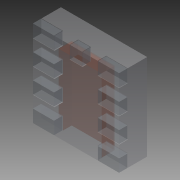
# Autodesk Inventor part: Si1143
Saved by Autodesk Inventor 2013 (Build 170138000, 138)
## iProperties
Created: 2015-06-30
Part Number: Si1143
Material: Ogólny
Document SubType Name: Modeling
Designer: terg
Density: 1 g/cm^3
Author: terg
Autodesk Inventor part; units mm, degrees
ref_plane "YZ Plane" through (0, 0, 0) normal (1, 0, 0) x (0, 1, 0)
ref_plane "XZ Plane" through (0, 0, 0) normal (0, 1, 0) x (-1, 0, 0)
sketch "Szkic1" plane through (0, 0, 0) normal (0, 1, 0) x (-1, 0, 0)
  line L0 (0, 0) -> (2, 0)
  line L1 (2, 0) -> (2, 2)
  line L2 (2, 2) -> (0, 2)
  line L3 (0, 2) -> (0, 0)
  dimension "d0" = 2
  dimension "d1" = 2
  constraints: 8 end point, 2 parallel, 1 horizontal, 1 perpendicular
  measures "d0" distance of L2.end L1.end
  measures "d1" distance of L1.end L0.end
extrude "Wyciągnięcie proste1" add sketch "Szkic1" along normal blind 0.65
sketch "Szkic2" plane through (0, 0, 0) normal (0, -1, 0) x (1, 0, 0)
  line L0 (0, 2) -> (0, 0) projected
  line L1 (-2, 2) -> (0, 2) projected
  line L2 (-2, 0) -> (-2, 2) projected
  line L3 (0, 0) -> (-0.5, 0)
  line L4 (-0.5, 0) -> (-0.5, 0.3)
  line L5 (-0.5, 0.3) -> (0, 0.3)
  line L6 (0, 0.3) -> (0, 0)
  line L7 (0, 0.5667) -> (-0.5, 0.5667)
  line L8 (-0.5, 0.5667) -> (-0.5, 0.8667)
  line L9 (-0.5, 0.8667) -> (0, 0.8667)
  line L10 (0, 0.8667) -> (0, 0.5667)
  line L11 (0, 1.1333) -> (-0.5, 1.1333)
  line L12 (-0.5, 1.1333) -> (-0.5, 1.4333)
  line L13 (-0.5, 1.4333) -> (0, 1.4333)
  line L14 (0, 1.4333) -> (0, 1.1333)
  line L15 (0, 1.7) -> (-0.5, 1.7)
  line L16 (-0.5, 1.7) -> (-0.5, 2)
  line L17 (-0.5, 2) -> (0, 2)
  line L18 (0, 2) -> (0, 1.7)
  line L19 (-2, 0) -> (-1.5, 0)
  line L20 (-1.5, 0) -> (-1.5, 0.3)
  line L21 (-1.5, 0.3) -> (-2, 0.3)
  line L22 (-2, 0.3) -> (-2, 0)
  line L23 (-2, 0.5667) -> (-1.5, 0.5667)
  line L24 (-1.5, 0.5667) -> (-1.5, 0.8667)
  line L25 (-1.5, 0.8667) -> (-2, 0.8667)
  line L26 (-2, 0.8667) -> (-2, 0.5667)
  line L27 (-2, 1.1333) -> (-1.5, 1.1333)
  line L28 (-1.5, 1.1333) -> (-1.5, 1.4333)
  line L29 (-1.5, 1.4333) -> (-2, 1.4333)
  line L30 (-2, 1.4333) -> (-2, 1.1333)
  line L31 (-2, 1.7) -> (-1.5, 1.7)
  line L32 (-1.5, 1.7) -> (-1.5, 2)
  line L33 (-1.5, 2) -> (-2, 2)
  line L34 (-2, 2) -> (-2, 1.7)
  line L35 (-0.85, 2) -> (-1.15, 2)
  line L36 (-1.15, 2) -> (-1.15, 1.7)
  line L37 (-1.15, 1.7) -> (-0.85, 1.7)
  line L38 (-0.85, 1.7) -> (-0.85, 2)
  dimension "d4" = 0.5
  dimension "d5" = 0.3
  dimension "d6" = 0.5
  dimension "d7" = 0.3
  dimension "d8" = 0.5
  dimension "d9" = 0.3
  dimension "d10" = 0.5
  dimension "d11" = 0.3
  dimension "d12" = 0
  dimension "d13" = 0.2667
  dimension "d14" = 0.2667
  dimension "d15" = 0.2667
  dimension "d16" = 0.5
  dimension "d17" = 0.3
  dimension "d18" = 0.5
  dimension "d19" = 0.3
  dimension "d20" = 0.5
  dimension "d21" = 0.3
  dimension "d22" = 0.5
  dimension "d23" = 0.3
  dimension "d24" = 0
  dimension "d25" = 0.2667
  dimension "d26" = 0.2667
  dimension "d27" = 0.3
  dimension "d28" = 0.3
  dimension "d29" = 0.85
  dimension "d30" = 0.85
  constraints: 72 end point, 19 equal length, 9 horizontal, 9 perpendicular, 7 point on line
  measures "d4" distance of L4.end L5.end
  measures "d5" distance of L3.end L4.end
  measures "d6" distance of L8.end L9.end
  measures "d7" distance of L7.end L8.end
  measures "d8" distance of L12.end L13.end
  measures "d9" distance of L11.end L12.end
  measures "d10" distance of L16.end L17.end
  measures "d11" distance of L15.end L16.end
  measures "d12" distance between parallel lines of L1 L17
  measures "d13" distance between parallel lines of L13 L15
  measures "d14" distance between parallel lines of L9 L11
  measures "d15" distance between parallel lines of L5 L7
  measures "d16" distance of L21.end L20.end
  measures "d17" distance of L20.end L19.end
  measures "d18" distance of L25.end L24.end
  measures "d19" distance of L24.end L23.end
  measures "d20" distance of L29.end L28.end
  measures "d21" distance of L28.end L27.end
  measures "d22" distance of L33.end L32.end
  measures "d23" distance of L32.end L31.end
  measures "d24" distance between parallel lines of L15 L31
  measures "d25" distance between parallel lines of L21 L23
  measures "d26" distance between parallel lines of L27 L25
  measures "d27" distance of L37.end L36.end
  measures "d28" distance of L36.end L35.end
  measures "d29" distance between parallel lines of L2 L36
  measures "d30" distance between parallel lines of L0 L38
extrude "Wyciągnięcie proste2" cut sketch "Szkic2" against normal blind 0.2
sketch "Szkic4" plane through (0, 0, 0) normal (0, -1, 0) x (1, 0, 0)
  line L0 (-1.5, 0.5667) -> (-2, 0.5667) projected
  line L1 (-2, 0.3) -> (-2, 0.5667) projected
  line L2 (-2, 0.3) -> (-1.5, 0.3) projected
  line L3 (-1.5, 0.3) -> (-1.5, 0) projected
  line L4 (-0.5, 0) -> (-1.5, 0) projected
  line L5 (-0.5, 0) -> (-0.5, 0.3) projected
  line L6 (-0.5, 0.3) -> (0, 0.3) projected
  line L7 (0, 0.5667) -> (-0.5, 0.5667) projected
  line L8 (-0.5, 0.5667) -> (-0.5, 0.8667) projected
  line L9 (-0.5, 0.8667) -> (0, 0.8667) projected
  line L10 (0, 1.1333) -> (-0.5, 1.1333) projected
  line L11 (-0.5, 1.1333) -> (-0.5, 1.4333) projected
  line L12 (-0.5, 1.4333) -> (0, 1.4333) projected
  line L13 (0, 1.7) -> (0, 1.4333) projected
  line L14 (0, 1.7) -> (-0.5, 1.7) projected
  line L15 (-0.5, 1.7) -> (-0.5, 2) projected
  line L16 (-0.85, 2) -> (-0.5, 2) projected
  line L17 (-0.85, 2) -> (-0.85, 1.7) projected
  line L18 (-0.85, 1.7) -> (-1.15, 1.7) projected
  line L19 (-1.15, 1.7) -> (-1.15, 2) projected
  line L20 (-1.5, 2) -> (-1.15, 2) projected
  line L21 (-1.5, 2) -> (-1.5, 1.7) projected
  line L22 (-1.5, 1.7) -> (-2, 1.7) projected
  line L23 (-2, 1.4333) -> (-2, 1.7) projected
  line L24 (-2, 1.4333) -> (-1.5, 1.4333) projected
  line L25 (-1.5, 1.4333) -> (-1.5, 1.1333) projected
  line L26 (-1.5, 1.1333) -> (-2, 1.1333) projected
  line L27 (-2, 0.8667) -> (-1.5, 0.8667) projected
  line L28 (-1.5, 0.8667) -> (-1.5, 0.5667) projected
  line L29 (-1.51, 1.71) -> (-2, 1.71)
  line L30 (-2, 1.71) -> (-2, 2)
  line L31 (-2, 2) -> (-1.51, 2)
  line L32 (-1.51, 2) -> (-1.51, 1.71)
  line L33 (-2, 1.4233) -> (-1.51, 1.4233)
  line L34 (-1.51, 1.4233) -> (-1.51, 1.1433)
  line L35 (-1.51, 1.1433) -> (-2, 1.1433)
  line L36 (-2, 1.1433) -> (-2, 1.4233)
  line L37 (-2, 0.8567) -> (-1.51, 0.8567)
  line L38 (-1.51, 0.8567) -> (-1.51, 0.5767)
  line L39 (-1.51, 0.5767) -> (-2, 0.5767)
  line L40 (-2, 0.5767) -> (-2, 0.8567)
  line L41 (-2, 0.29) -> (-1.51, 0.29)
  line L42 (-1.51, 0.29) -> (-1.51, 0)
  line L43 (-1.51, 0) -> (-2, 0)
  line L44 (-2, 0) -> (-2, 0.29)
  line L45 (-0.49, 0.29) -> (0, 0.29)
  line L46 (0, 0.29) -> (0, 0)
  line L47 (0, 0) -> (-0.49, 0)
  line L48 (-0.49, 0) -> (-0.49, 0.29)
  line L49 (-0.49, 0.8567) -> (0, 0.8567)
  line L50 (0, 0.8567) -> (0, 0.5767)
  line L51 (0, 0.5767) -> (-0.49, 0.5767)
  line L52 (-0.49, 0.5767) -> (-0.49, 0.8567)
  line L53 (-0.49, 1.4233) -> (0, 1.4233)
  line L54 (0, 1.4233) -> (0, 1.1433)
  line L55 (0, 1.1433) -> (-0.49, 1.1433)
  line L56 (-0.49, 1.1433) -> (-0.49, 1.4233)
  line L57 (-0.49, 2) -> (0, 2)
  line L58 (0, 2) -> (0, 1.71)
  line L59 (0, 1.71) -> (-0.49, 1.71)
  line L60 (-0.49, 1.71) -> (-0.49, 2)
  line L61 (-1.14, 2) -> (-0.86, 2)
  line L62 (-0.86, 2) -> (-0.86, 1.71)
  line L63 (-0.86, 1.71) -> (-1.14, 1.71)
  line L64 (-1.14, 1.71) -> (-1.14, 2)
  dimension "d33" = 0.01
  dimension "d34" = 0.01
  dimension "d35" = 0
  dimension "d36" = 0
  dimension "d37" = 0.01
  dimension "d38" = 0.01
  dimension "d39" = 0.01
  dimension "d40" = 0
  dimension "d41" = 0.01
  dimension "d42" = 0.01
  dimension "d43" = 0
  dimension "d44" = 0.01
  dimension "d45" = 0.01
  dimension "d46" = 0.01
  dimension "d47" = 0.01
  dimension "d48" = 0.01
  dimension "d49" = 0.01
  dimension "d50" = 0.01
  dimension "d51" = 0.01
  dimension "d52" = 0
  dimension "d53" = 0
  dimension "d54" = 0.01
  dimension "d55" = 0.01
  dimension "d56" = 0.01
  dimension "d57" = 0.01
  dimension "d58" = 0.01
  dimension "d59" = 0.01
  dimension "d60" = 0.01
  dimension "d61" = 0.01
  constraints: 72 end point, 18 parallel, 9 horizontal, 9 perpendicular, 1 collinear
  measures "d33" distance between parallel lines of L21 L32
  measures "d34" distance between parallel lines of L22 L29
  measures "d35" distance between parallel lines of L20 L31
  measures "d36" distance between parallel lines of L23 L30
  measures "d37" distance between parallel lines of L19 L64
  measures "d38" distance between parallel lines of L17 L62
  measures "d39" distance between parallel lines of L18 L63
  measures "d40" distance between parallel lines of L16 L57
  measures "d41" distance between parallel lines of L15 L60
  measures "d42" distance between parallel lines of L14 L59
  measures "d43" distance between parallel lines of L13 L58
  measures "d44" distance between parallel lines of L24 L33
  measures "d45" distance between parallel lines of L25 L34
  measures "d46" distance between parallel lines of L26 L35
  measures "d47" distance between parallel lines of L27 L37
  measures "d48" distance between parallel lines of L0 L39
  measures "d49" distance between parallel lines of L28 L38
  measures "d50" distance between parallel lines of L3 L42
  measures "d51" distance between parallel lines of L2 L41
  measures "d52" distance between parallel lines of L1 L44
  measures "d53" distance between parallel lines of L4 L43
  measures "d54" distance between parallel lines of L5 L48
  measures "d55" distance between parallel lines of L6 L45
  measures "d56" distance between parallel lines of L7 L51
  measures "d57" distance between parallel lines of L9 L49
  measures "d58" distance between parallel lines of L8 L52
  measures "d59" distance between parallel lines of L10 L55
  measures "d60" distance between parallel lines of L11 L56
  measures "d61" distance between parallel lines of L12 L53
extrude "Wyciągnięcie proste3" add sketch "Szkic4" against normal blind 0.19
ref_plane "Płaszczyzna konstrukcyjna1" through (0, 0.2, 0) normal (0, 1, 0) x (1, 0, 0)
sketch "Szkic5" plane through (0, 0.2, 0) normal (0, 1, 0) x (1, 0, 0)
  line L0 (-1.5, 0) -> (-0.5, 0)
  line L1 (-0.5, 0) -> (-0.5, -1.7)
  line L2 (-0.5, -1.7) -> (-1.5, -1.7)
  line L3 (-1.5, -1.7) -> (-1.5, 0)
  line L4 (0, -2) -> (0, 0) projected
  line L5 (-2, 0) -> (-2, -2) projected
  line L6 (0, 0) -> (-2, 0) projected
  dimension "d65" = 1
  dimension "d66" = 1.7
  dimension "d67" = 0.5
  dimension "d68" = 0.5
  dimension "d69" = 0
  constraints: 8 end point, 2 parallel, 1 horizontal, 1 perpendicular
  measures "d65" distance of L1.end L2.end
  measures "d66" distance of L0.end L1.end
  measures "d67" distance between parallel lines of L4 L1
  measures "d68" distance between parallel lines of L5 L3
  measures "d69" distance between parallel lines of L6 L0
extrude "Wyciągnięcie proste4" cut sketch "Szkic5" along normal blind 0.2 and the other way blind 0.1
sketch "Szkic7" plane through (0, 0.1, 0) normal (0, 1, 0) x (1, 0, 0)
  line L0 (-1.5, 0) -> (-0.5, 0) projected
  line L1 (-0.505, 0) -> (-1.495, 0)
  line L2 (-1.495, 0) -> (-1.495, -1.69)
  line L3 (-1.495, -1.69) -> (-0.505, -1.69)
  line L4 (-0.505, -1.69) -> (-0.505, 0)
  line L5 (0, -2) -> (0, 0) projected
  line L6 (-2, 0) -> (-2, -2) projected
  dimension "d81" = 0.99
  dimension "d82" = 1.69
  dimension "d83" = 0.505
  dimension "d84" = 0.505
  constraints: 8 end point, 2 parallel, 1 horizontal, 1 perpendicular, 1 point on line
  measures "d81" distance of L3.end L2.end
  measures "d82" distance of L2.end L1.end
  measures "d83" distance between parallel lines of L5 L4
  measures "d84" distance between parallel lines of L6 L2
extrude "Wyciągnięcie proste6" add sketch "Szkic7" along normal blind 0.28
equation "\"d6\" = d4"
equation "\"d7\" = d5"
equation "\"d8\" = d4"
equation "\"d9\" = d5"
equation "\"d10\" = d4"
equation "\"d11\" = d5"
equation "\"d13\" = d14"
equation "\"d14\" = d15"
equation "\"d16\" = d4"
equation "\"d17\" = d5"
equation "\"d18\" = d4"
equation "\"d19\" = d5"
equation "\"d20\" = d4"
equation "\"d21\" = d5"
equation "\"d23\" = d5"
equation "\"d25\" = d15"
equation "\"d26\" = d15"
equation "\"d29\" = d30"
equation "\"d33\" = d34"
equation "\"d37\" = d34"
equation "\"d38\" = d34"
equation "\"d39\" = d34"
equation "\"d41\" = d34"
equation "\"d42\" = d34"
equation "\"d44\" = d34"
equation "\"d45\" = d34"
equation "\"d46\" = d34"
equation "\"d47\" = d34"
equation "\"d48\" = d34"
equation "\"d49\" = d34"
equation "\"d50\" = d34"
equation "\"d51\" = d34"
equation "\"d54\" = d34"
equation "\"d55\" = d34"
equation "\"d56\" = d34"
equation "\"d57\" = d34"
equation "\"d58\" = d34"
equation "\"d59\" = d34"
equation "\"d60\" = d34"
equation "\"d61\" = d34"
equation "\"d67\" = d68"
equation "\"d83\" = d84"
